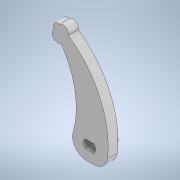
# Autodesk Inventor part: mavac_ruka I guesss
Saved by Autodesk Inventor 2022 (Build 260153000, 153)
## iProperties
Created: 2022-08-25
Part Number: mavac_ruka I guesss
Material: Generic
Document SubType Name: Modeling
Designer: Ruslana Zubareva
Density: 1 g/cm^3
Appearance: Default
Author: Ruslana Zubareva
Autodesk Inventor part; units mm, degrees
ref_plane "YZ Plane" through (0, 0, 0) normal (1, 0, 0) x (0, 1, 0)
ref_plane "XZ Plane" through (0, 0, 0) normal (0, 1, 0) x (-1, 0, 0)
ref_plane "XY Plane" through (0, 0, 0) normal (0, 0, 1) x (1, 0, 0)
sketch "Sketch1" plane through (0, 0, 0) normal (0, 0, 1) x (1, 0, 0)
  arc A0 (6.3455, 7.6592) -> (2.9969, 4.161) centre (5.1207, 5.4798) ccw
  arc A1 (28.9309, -45.2636) -> (10.279, 5.1864) centre (-16.779, -33.4901) ccw
  arc A2 (8.9309, -45.2636) -> (6.4804, -0.2246) centre (-28.4708, -24.7125) ccw
  line L0 (8.9309, -45.2636) -> (28.9309, -45.2636)
  line L1 (22.9916, -36.6135) -> (18.8703, -36.6135)
  line L2 (22.9916, -39.6135) -> (18.8703, -39.6135)
  line L3 (20.9309, -34.0784) -> (20.9309, -41.4431) construction
  line L4 (22.8639, -38.1135) -> (15.5009, -38.1135) construction
  arc A3 (18.8703, -36.6135) -> (18.8703, -39.6135) centre (20.9309, -38.1135) ccw
  arc A4 (22.9916, -39.6135) -> (22.9916, -36.6135) centre (20.9309, -38.1135) ccw
  line L5 (18.6071, -36.0635) -> (23.2547, -36.0635)
  arc A5 (23.2547, -40.1635) -> (23.2547, -36.0635) centre (20.9309, -38.1135) ccw
  line L6 (23.2547, -40.1635) -> (18.6071, -40.1635)
  arc A6 (18.6071, -36.0635) -> (18.6071, -40.1635) centre (20.9309, -38.1135) ccw
  arc A7 (2.9969, 4.161) -> (6.4804, -0.2246) centre (4.7985, 2.0157) ccw
  arc A8 (10.279, 5.1864) -> (5.805, 7.8843) centre (7.5999, 5.8022) ccw
  point P0 (0, 0)
  dimension "d25" = 2.5
  dimension "d32" = 20
  dimension "d40" = 1.5
  dimension "d41" = 1.5
  dimension "d42" = 8
  dimension "d43" = 7.1502
  dimension "d44" = 0.55
  constraints: 20 point on circle, 14 end point, 9 centre point, 3 horizontal, 2 parallel, 1 point on line, 1 tangent, 1 vertical, 3 other
  measures "d25" radius of A0
  measures "d32" distance of L0.start L0.end
  measures "d40" distance from line of L1 A3.centre
  measures "d41" distance from line of A3.centre L2
  measures "d42" horizontal distance of L0.end A3.centre
  measures "d43" distance from line of L0 A3.centre
  measures "d44" distance between parallel lines of L1 L5
extrude "Extrusion1" add sketch "Sketch1" along normal blind 5 contours A8 A1 L0 A2 A7 A0
sketch "Sketch3" plane through (0, 0, 0) normal (0, 0, -1) x (-1, 0, 0)
  line L0 (-18.6071, -36.0635) -> (-23.2547, -36.0635) projected
  arc A0 (-23.2547, -36.0635) -> (-23.2547, -40.1635) centre (-20.9309, -38.1135) ccw projected
  line L1 (-23.2547, -40.1635) -> (-18.6071, -40.1635) projected
  arc A1 (-18.6071, -40.1635) -> (-18.6071, -36.0635) centre (-20.9309, -38.1135) ccw projected
  line L2 (-23.8543, -34.5635) -> (-18.0075, -34.5635)
  arc A2 (-18.0075, -41.6635) -> (-18.0075, -34.5635) centre (-20.9309, -38.1135) ccw
  line L3 (-18.0075, -41.6635) -> (-23.8543, -41.6635)
  arc A3 (-23.8543, -34.5635) -> (-23.8543, -41.6635) centre (-20.9309, -38.1135) ccw
  point P0 (0, 0)
  dimension "d45" = 1.5
  constraints: 4 end point, 4 point on circle, 2 centre point, 3 other
  measures "d45" distance between parallel lines of L0 L2
extrude "Extrusion3" add sketch "Sketch3" along normal blind 5
fillet "Fillet2" radius 7 2 edges at (8.9309, -45.2636, 2.5) (28.9309, -45.2636, 2.5)
body "Solid1"
